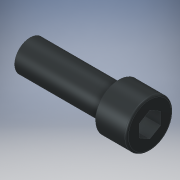
# Autodesk Inventor part: M3.5
Saved by Autodesk Inventor 2019 (Build 230136000, 136)
## iProperties
Created: 2020-02-22
Part Number: M3.5
Material: Iron, Cast
Document SubType Name: Modeling
Designer: Elías Sánchez
Density: 7.15 g/cm^3
Appearance: Iron Gray
Author: Elías Sánchez
Autodesk Inventor part; units mm, degrees
ref_plane "YZ Plane" through (0, 0, 0) normal (1, 0, 0) x (0, 1, 0)
ref_plane "XZ Plane" through (0, 0, 0) normal (0, 1, 0) x (-1, 0, 0)
ref_plane "XY Plane" through (0, 0, 0) normal (0, 0, 1) x (1, 0, 0)
sketch "Sketch1" plane through (0, 0, 0) normal (1, 0, 0) x (0, 1, 0)
  circle A0 centre (0, 0) radius 1.75
  dimension "d0" = 3.5
  constraints: 1 centre point, 1 coincident
  measures "d0" diameter of A0
extrude "Extrusion1" add sketch "Sketch1" along normal blind 10
sketch "Sketch2" plane through (10, 0, 0) normal (1, 0, 0) x (0, 0, -1)
  circle A0 centre (0, 0) radius 2.625
  dimension "d3" = 5.25
  constraints: 1 centre point, 1 coincident
  measures "d3" diameter of A0
extrude "Extrusion2" add sketch "Sketch2" along normal blind 3.5
ref_plane "Work Plane1" through (13.5, 0, 0) normal (1, 0, 0) x (0, 0, -1)
sketch "Sketch3" plane through (13.5, 0, 0) normal (1, 0, 0) x (0, 0, -1)
  line L0 (0, -1.4) -> (-1.2124, -0.7)
  line L1 (-1.2124, -0.7) -> (-1.2124, 0.7)
  line L2 (-1.2124, 0.7) -> (0, 1.4)
  line L3 (0, 1.4) -> (1.2124, 0.7)
  line L4 (1.2124, 0.7) -> (1.2124, -0.7)
  line L5 (1.2124, -0.7) -> (0, -1.4)
  point P0 (0, 0)
  point P1 (0, 0)
  dimension "d9" = 2.8
  dimension "d10" = 1.2124
  constraints: 12 end point, 1 coincident, 13 other
  measures "d9" distance of L0.start L2.end
  measures "d10" horizontal distance of L4.end L0.start
extrude "Extrusion3" cut sketch "Sketch3" against normal blind 1.75
fillet "Fillet2" radius 0.2 1 edges at (13.5, 0, 2.625)
body "Solid1"
